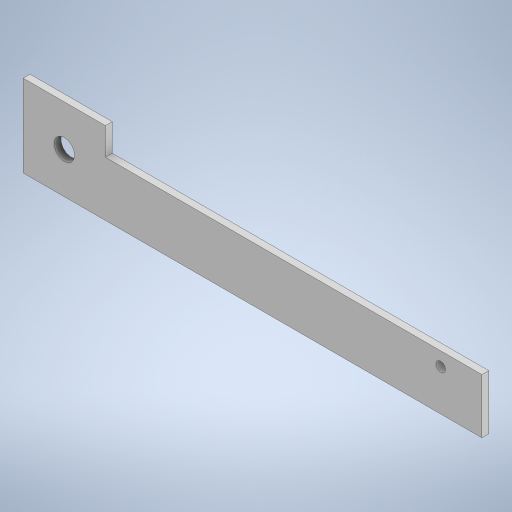
# Autodesk Inventor part: conveyor belt sideplank
Saved by Autodesk Inventor 2023 (Build 270158000, 158)
## iProperties
Created: 2022-06-04
Part Number: conveyor belt sideplank
Material: Generic
Document SubType Name: Modeling
Designer: prana_p9lsmih
Density: 1 g/cm^3
Appearance: Default
Author: prana_p9lsmih
Autodesk Inventor part; units mm, degrees
ref_plane "YZ Plane" through (0, 0, 0) normal (1, 0, 0) x (0, 1, 0)
ref_plane "XZ Plane" through (0, 0, 0) normal (0, 1, 0) x (-1, 0, 0)
ref_plane "XY Plane" through (0, 0, 0) normal (0, 0, 1) x (1, 0, 0)
sketch "Sketch11" plane through (0, 0, 0) normal (0, 0, 1) x (1, 0, 0)
  line L0 (0, 0) -> (335, 0)
  line L1 (0, 0) -> (0, 60)
  line L2 (0, 60) -> (60, 60)
  line L3 (60, 60) -> (60, 40)
  line L4 (275, 40) -> (60, 40)
  circle A0 centre (30, 30) radius 7.5
  circle A1 centre (305, 30) radius 3.5
  line L5 (275, 40) -> (335, 40)
  line L6 (335, 40) -> (335, 0)
  dimension "d110" = 60
  dimension "d111" = 60
  dimension "d112" = 20
  dimension "d114" = 15
  dimension "d115" = 7
  dimension "d120" = 60
  constraints: 14 end point, 3 horizontal, 2 centre point, 2 perpendicular, 1 vertical
  measures "d110" distance of L0.start L1.end
  measures "d111" distance of L1.end L2.end
  measures "d112" distance of L2.end L3.end
  measures "d114" diameter of A0
  measures "d115" diameter of A1
  measures "d120" distance of L4.start L5.end
extrude "Extrusion2" add sketch "Sketch11" along normal blind 5
body "Solid2"
